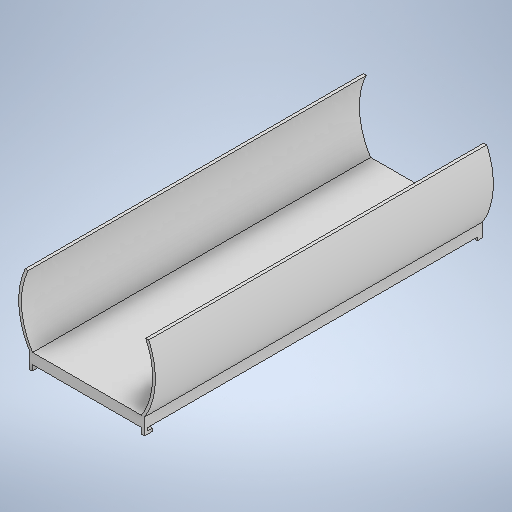
# Autodesk Inventor part: PCB Battery Tray
Saved by Autodesk Inventor 2025 (Build 290162000, 162)
## iProperties
Created: 2024-07-12
Part Number: PCB Battery Tray
Material: Generic
Document SubType Name: Modeling
Designer: track
Density: 1 g/cm^3
Appearance: Default
Author: track
## iProperties of the stored document PCB Battery Tray_3DPrint.ipt
Created: 2024-07-12
Part Number: PCB Battery Tray_3DPrint
Material: Generic
Document SubType Name: Modeling
Designer: track
Density: 1 g/cm^3
Appearance: Default
Author: track
Autodesk Inventor part; units mm, degrees
ref_plane "YZ Plane" through (0, 0, 0) normal (1, 0, 0) x (0, 1, 0)
ref_plane "XZ Plane" through (0, 0, 0) normal (0, 1, 0) x (-1, 0, 0)
ref_plane "XY Plane" through (0, 0, 0) normal (0, 0, 1) x (1, 0, 0)
sketch "Sketch1" plane through (0, 0, 0) normal (0, 0, 1) x (1, 0, 0)
  line L0 (0, 0) -> (0, 2.54)
  line L1 (0, 2.54) -> (35.6964, 2.54)
  line L2 (35.6964, 2.54) -> (35.6964, 0)
  line L3 (-0.889, 0) -> (-0.889, 3.429)
  line L4 (-0.889, 3.429) -> (36.5854, 3.429)
  line L5 (36.5854, 3.429) -> (36.5854, 0)
  line L6 (-0.889, 0) -> (0, 0)
  line L7 (35.6964, 0) -> (36.5854, 0)
  line L8 (33.7232, 32.179) -> (1.9732, 32.179)
  arc A0 (36.5854, 3.429) -> (33.7232, 32.179) centre (16.0324, 15.9003) ccw
  line L9 (17.8482, 3.429) -> (17.8482, 32.179) construction
  arc A1 (1.9732, 32.179) -> (-0.889, 3.429) centre (19.664, 15.9003) ccw
  line L10 (40.0732, 15.9003) -> (-4.3768, 15.9003)
  arc A2 (35.5381, 3.429) -> (33.3287, 31.29) centre (16.0324, 15.9003) ccw
  line L11 (33.3287, 31.29) -> (2.3677, 31.29)
  arc A3 (2.3677, 31.29) -> (0.1583, 3.429) centre (19.664, 15.9003) ccw
  dimension "d0" = 35.6964
  dimension "d1" = 2.54
  dimension "d2" = 2.54
  dimension "d3" = 0.889
  dimension "d11" = 28.75
  dimension "d14" = 31.75
  dimension "d15" = 0
  dimension "d16" = 44.45
  dimension "d17" = 0.889
  constraints: 24 end point, 10 point on circle, 4 centre point, 4 perpendicular, 3 horizontal, 2 midpoint, 2 point on line, 1 collinear, 1 vertical, 5 other
  measures "d0" distance of L0.end L1.end
  measures "d1" distance of L1.end L2.end
  measures "d2" distance of L0.start L0.end
  measures "d3" distance between parallel lines of L3 L0
  measures "d11" distance between parallel lines of L4 L8
  measures "d14" distance of L8.start L8.end
  measures "d15" distance from line of A0.centre L10
  measures "d16" distance of L10.start L10.end
  measures "d17" radial gap between concentric circles of A0 A2
extrude "Extrusion1" add sketch "Sketch1" against normal blind 110 contours L6 L3 L4 L5 L7 L2 L1 L0 | A1 L10 A3 L4 | A1 L8 A0 L10 A2 L11 A3 | A2 L10 A0 L4
sketch "Sketch2" plane through (0, 0, 0) normal (0, 0, 1) x (1, 0, 0)
  line L0 (-0.889, 3.429) -> (36.5854, 3.429)
  line L1 (36.5854, 3.429) -> (36.5854, 0)
  line L2 (36.5854, 0) -> (-0.889, 0)
  line L3 (-0.889, 0) -> (-0.889, 3.429)
  line L4 (36.5854, 0) -> (36.5854, 3.429) projected
  line L5 (35.6964, 0) -> (36.5854, 0) projected
  line L6 (35.5381, 3.429) -> (0.1583, 3.429) projected
  line L7 (-0.889, 3.429) -> (-0.889, 0) projected
  constraints: 8 end point, 4 collinear, 2 parallel, 1 horizontal, 1 perpendicular
extrude "Extrusion2" add sketch "Sketch2" against normal blind 1
sketch "Sketch3" plane through (0, 0, -110) normal (0, 0, -1) x (-1, 0, 0)
  arc A0 (-33.7232, 32.179) -> (-36.5854, 3.429) centre (-16.0324, 15.9003) ccw projected
  line L0 (-37.9272, 25.829) -> (2.2308, 25.829)
  line L1 (2.2308, 25.829) -> (2.2308, 32.179)
  line L2 (2.2308, 32.179) -> (-37.9272, 32.179)
  line L3 (-37.9272, 32.179) -> (-37.9272, 25.829)
  line L4 (-1.9732, 32.179) -> (-33.7232, 32.179) projected
  line L5 (-17.8482, 32.179) -> (-17.8482, 3.429)
  line L6 (-35.5381, 3.429) -> (-0.1583, 3.429) projected
  point P0 (0, 0)
  dimension "d18" = 0
  dimension "d19" = 6.35
  constraints: 10 end point, 2 midpoint, 2 parallel, 1 horizontal, 1 perpendicular, 1 point on circle, 1 vertical, 1 other
  measures "d18" distance between parallel lines of L4 L2
  measures "d19" distance of L2.end L0.start
extrude "Extrusion3" cut sketch "Sketch3" against normal through all contours L2 L5 L0 A0 | L2 L1 L0 L5
sketch "Sketch4" plane through (0, 0, 0) normal (0, 0, 1) x (1, 0, 0)
  line L0 (35.6964, 0) -> (35.6964, 2.54) projected
  line L1 (35.6964, 0) -> (36.5854, 0)
  line L2 (36.5854, 0) -> (36.5854, -0.889)
  line L3 (36.5854, -0.889) -> (35.6964, -0.889)
  line L4 (35.6964, -0.889) -> (35.6964, 0)
  line L5 (36.5854, 0) -> (36.5854, 3.429) projected
  line L6 (0, 0) -> (-0.889, 0)
  line L7 (-0.889, 0) -> (-0.889, -0.889)
  line L8 (-0.889, -0.889) -> (0, -0.889)
  line L9 (0, -0.889) -> (0, 0)
  line L10 (-0.889, 3.429) -> (-0.889, 0) projected
  dimension "d23" = 0.889
  dimension "d24" = 0.889
  constraints: 16 end point, 4 parallel, 2 collinear, 2 horizontal, 2 perpendicular
  measures "d23" distance of L1.end L2.end
  measures "d24" distance of L8.end L6.start
extrude "Extrusion4" add sketch "Sketch4" against normal blind 1
sketch "Sketch5" plane through (-0.889, -0.889, 0) normal (0, -1, 0) x (1, 0, 0)
  line L0 (0.889, 0) -> (0.889, -1) projected
  line L1 (0, -1) -> (0, -110) projected
  line L2 (0.889, 0) -> (0, 0)
  line L3 (0, 0) -> (0, -2.54)
  line L4 (0, -2.54) -> (0.889, -2.54)
  line L5 (0.889, -2.54) -> (0.889, 0)
  line L6 (37.4744, 0) -> (37.4744, -110) projected
  line L7 (37.4744, 0) -> (36.5854, 0)
  line L8 (36.5854, 0) -> (36.5854, -2.54)
  line L9 (36.5854, -2.54) -> (37.4744, -2.54)
  line L10 (37.4744, -2.54) -> (37.4744, 0)
  line L11 (36.5854, -1) -> (36.5854, -110) projected
  dimension "d27" = 2.54
  dimension "d28" = 2.54
  constraints: 16 end point, 4 parallel, 2 horizontal, 2 perpendicular, 1 collinear, 1 point on line
  measures "d27" distance of L4.end L0.start
  measures "d28" distance of L7.end L8.end
extrude "Extrusion5" add sketch "Sketch5" along normal blind 1
sketch "Sketch6" plane through (35.6964, 0, -110) normal (0, -1, 0) x (1, 0, 0)
  line L0 (0.889, 110) -> (0.889, 0) projected
  line L1 (0, 109) -> (0, 0) projected
  line L2 (0.889, 0) -> (0, 0)
  line L3 (0, 0) -> (0, 1.651)
  line L4 (0, 1.651) -> (0.889, 1.651)
  line L5 (0.889, 1.651) -> (0.889, 0)
  line L6 (-36.5854, 109) -> (-36.5854, 0) projected
  line L7 (-35.6964, 109) -> (-35.6964, 0) projected
  line L8 (-36.5854, 0) -> (-35.6964, 0)
  line L9 (-35.6964, 0) -> (-35.6964, 1.651)
  line L10 (-35.6964, 1.651) -> (-36.5854, 1.651)
  line L11 (-36.5854, 1.651) -> (-36.5854, 0)
  point P0 (-35.6964, 110)
  point P1 (-36.5854, 1.651)
  point P2 (0.889, 1.651)
  dimension "d31" = 1.651
  dimension "d32" = 1.651
  constraints: 16 end point, 4 parallel, 2 horizontal, 2 perpendicular, 2 point on line
  measures "d31" distance between parallel lines of L4 L2
  measures "d32" distance between parallel lines of L8 L10
extrude "Extrusion6" add sketch "Sketch6" along normal blind 1
body "Solid1"
